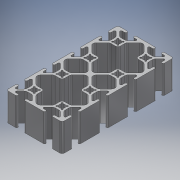
# Autodesk Inventor part: 2040-S
Saved by Autodesk Inventor 2017 SP1 (Build 210196100, 196)
## iProperties
Created: 2016-09-13
Part Number: 2040-S
Material: 6105-T5
Description: 40 S SHORT SINGLE UNIBEARING ASSEMBLY ON 40-4040 X 75mm
Document SubType Name: Modeling
Designer: BRALEF
Density: 1 g/cm^3
Appearance: CLEAR ANODIZED
MATERIAL: 6061-T6
PART PRICE: 44.65
Author: BRALEF
Autodesk Inventor part; units mm, degrees
ref_plane "YZ Plane" through (0, 0, 0) normal (1, 0, 0) x (0, 1, 0)
ref_plane "XZ Plane" through (0, 0, 0) normal (0, 1, 0) x (-1, 0, 0)
ref_plane "XY Plane" through (0, 0, 0) normal (0, 0, 1) x (1, 0, 0)
sketch "Sketch1" plane through (0, 0, 0) normal (0, 1, 0) x (-1, 0, 0)
  arc A0 (-10.6413, -41.7213) -> (-14.7587, -41.7213) centre (-12.7, -43.78) ccw
  line L0 (-19.9529, -46.9156) -> (-14.7587, -41.7213)
  arc A1 (-19.9529, -46.9156) -> (-20.8828, -49.1606) centre (-17.7078, -49.1606) ccw
  line L1 (-20.8828, -53.1074) -> (-20.8828, -49.1606)
  arc A2 (-23.0926, -55.3172) -> (-20.8828, -53.1074) centre (-23.0926, -53.1074) ccw
  line L2 (-27.0394, -55.3172) -> (-23.0926, -55.3172)
  arc A3 (-27.0394, -55.3172) -> (-29.2844, -56.2471) centre (-27.0394, -58.4922) ccw
  line L3 (-34.4787, -61.4413) -> (-29.2844, -56.2471)
  arc A4 (-34.4787, -61.4413) -> (-34.4787, -65.5587) centre (-32.42, -63.5) ccw
  line L4 (-29.2844, -70.7529) -> (-34.4787, -65.5587)
  arc A5 (-29.2844, -70.7529) -> (-27.0394, -71.6828) centre (-27.0394, -68.5078) ccw
  line L5 (-23.0926, -71.6828) -> (-27.0394, -71.6828)
  arc A6 (-20.8828, -73.8926) -> (-23.0926, -71.6828) centre (-23.0926, -73.8926) ccw
  line L6 (-20.8828, -77.8394) -> (-20.8828, -73.8926)
  arc A7 (-20.8828, -77.8394) -> (-19.9529, -80.0844) centre (-17.7078, -77.8394) ccw
  line L7 (-14.7587, -85.2787) -> (-19.9529, -80.0844)
  arc A8 (-14.7587, -85.2787) -> (-10.6413, -85.2787) centre (-12.7, -83.22) ccw
  line L8 (-5.4471, -80.0844) -> (-10.6413, -85.2787)
  arc A9 (-5.4471, -80.0844) -> (-4.5172, -77.8394) centre (-7.6922, -77.8394) ccw
  line L9 (-4.5172, -73.8926) -> (-4.5172, -77.8394)
  arc A10 (-2.3074, -71.6828) -> (-4.5172, -73.8926) centre (-2.3074, -73.8926) ccw
  line L10 (1.6394, -71.6828) -> (-2.3074, -71.6828)
  arc A11 (1.6394, -71.6828) -> (3.8844, -70.7529) centre (1.6394, -68.5078) ccw
  line L11 (9.0787, -65.5587) -> (3.8844, -70.7529)
  arc A12 (9.0787, -65.5587) -> (9.0787, -61.4413) centre (7.02, -63.5) ccw
  line L12 (3.8844, -56.2471) -> (9.0787, -61.4413)
  arc A13 (3.8844, -56.2471) -> (1.6394, -55.3172) centre (1.6394, -58.4922) ccw
  line L13 (-2.3074, -55.3172) -> (1.6394, -55.3172)
  arc A14 (-4.5172, -53.1074) -> (-2.3074, -55.3172) centre (-2.3074, -53.1074) ccw
  line L14 (-4.5172, -49.1606) -> (-4.5172, -53.1074)
  arc A15 (-4.5172, -49.1606) -> (-5.4471, -46.9156) centre (-7.6922, -49.1606) ccw
  line L15 (-10.6413, -41.7213) -> (-5.4471, -46.9156)
  arc A16 (-9.0785, -36.041) -> (-9.0785, -40.159) centre (-7.0195, -38.1) ccw
  line L16 (-3.8846, -45.3529) -> (-9.0785, -40.159)
  arc A17 (-3.8846, -45.3529) -> (-1.6396, -46.2828) centre (-1.6396, -43.1078) ccw
  line L17 (1.6396, -46.2828) -> (-1.6396, -46.2828)
  arc A18 (1.6396, -46.2828) -> (3.8846, -45.3529) centre (1.6396, -43.1078) ccw
  line L18 (9.0785, -40.159) -> (3.8846, -45.3529)
  arc A19 (9.0785, -40.159) -> (9.0785, -36.041) centre (7.0195, -38.1) ccw
  line L19 (3.8846, -30.8471) -> (9.0785, -36.041)
  arc A20 (3.8846, -30.8471) -> (1.6396, -29.9172) centre (1.6396, -33.0922) ccw
  line L20 (-1.6396, -29.9172) -> (1.6396, -29.9172)
  arc A21 (-1.6396, -29.9172) -> (-3.8846, -30.8471) centre (-1.6396, -33.0922) ccw
  line L21 (-9.0785, -36.041) -> (-3.8846, -30.8471)
  arc A22 (-27.3692, -73.3395) -> (-28.2605, -74.2308) centre (-27.8696, -73.7304) ccw
  line L22 (-27.6319, -74.8595) -> (-28.2605, -74.2308)
  arc A23 (-27.6319, -74.8595) -> (-27.6319, -77.5405) centre (-25.4, -76.2) ccw
  line L23 (-28.2605, -78.1692) -> (-27.6319, -77.5405)
  arc A24 (-28.2605, -78.1692) -> (-27.3692, -79.0605) centre (-27.8696, -78.6696) ccw
  line L24 (-26.7405, -78.4319) -> (-27.3692, -79.0605)
  arc A25 (-26.7405, -78.4319) -> (-24.0595, -78.4319) centre (-25.4, -76.2) ccw
  line L25 (-23.4308, -79.0605) -> (-24.0595, -78.4319)
  arc A26 (-23.4308, -79.0605) -> (-22.5395, -78.1692) centre (-22.9304, -78.6696) ccw
  line L26 (-23.1681, -77.5405) -> (-22.5395, -78.1692)
  arc A27 (-23.1681, -77.5405) -> (-23.1681, -74.8595) centre (-25.4, -76.2) ccw
  line L27 (-22.5395, -74.2308) -> (-23.1681, -74.8595)
  arc A28 (-22.5395, -74.2308) -> (-23.4308, -73.3395) centre (-22.9304, -73.7304) ccw
  line L28 (-24.0595, -73.9681) -> (-23.4308, -73.3395)
  arc A29 (-24.0595, -73.9681) -> (-26.7405, -73.9681) centre (-25.4, -76.2) ccw
  line L29 (-27.3692, -73.3395) -> (-26.7405, -73.9681)
  arc A30 (-27.3692, -47.9395) -> (-28.2605, -48.8308) centre (-27.8696, -48.3304) ccw
  line L30 (-27.6319, -49.4595) -> (-28.2605, -48.8308)
  arc A31 (-27.6319, -49.4595) -> (-27.6319, -52.1405) centre (-25.4, -50.8) ccw
  line L31 (-28.2605, -52.7692) -> (-27.6319, -52.1405)
  arc A32 (-28.2605, -52.7692) -> (-27.3692, -53.6605) centre (-27.8696, -53.2696) ccw
  line L32 (-26.7405, -53.0319) -> (-27.3692, -53.6605)
  arc A33 (-26.7405, -53.0319) -> (-24.0595, -53.0319) centre (-25.4, -50.8) ccw
  line L33 (-23.4308, -53.6605) -> (-24.0595, -53.0319)
  arc A34 (-23.4308, -53.6605) -> (-22.5395, -52.7692) centre (-22.9304, -53.2696) ccw
  line L34 (-23.1681, -52.1405) -> (-22.5395, -52.7692)
  arc A35 (-23.1681, -52.1405) -> (-23.1681, -49.4595) centre (-25.4, -50.8) ccw
  line L35 (-22.5395, -48.8308) -> (-23.1681, -49.4595)
  arc A36 (-22.5395, -48.8308) -> (-23.4308, -47.9395) centre (-22.9304, -48.3304) ccw
  line L36 (-24.0595, -48.5681) -> (-23.4308, -47.9395)
  arc A37 (-24.0595, -48.5681) -> (-26.7405, -48.5681) centre (-25.4, -50.8) ccw
  line L37 (-27.3692, -47.9395) -> (-26.7405, -48.5681)
  arc A38 (-1.9692, -22.5395) -> (-2.8605, -23.4308) centre (-2.4696, -22.9304) ccw
  line L38 (-2.2319, -24.0595) -> (-2.8605, -23.4308)
  arc A39 (-2.2319, -24.0595) -> (-2.2319, -26.7405) centre (0, -25.4) ccw
  line L39 (-2.8605, -27.3692) -> (-2.2319, -26.7405)
  arc A40 (-2.8605, -27.3692) -> (-1.9692, -28.2605) centre (-2.4696, -27.8696) ccw
  line L40 (-1.3405, -27.6319) -> (-1.9692, -28.2605)
  arc A41 (-1.3405, -27.6319) -> (1.3405, -27.6319) centre (0, -25.4) ccw
  line L41 (1.9692, -28.2605) -> (1.3405, -27.6319)
  arc A42 (1.9692, -28.2605) -> (2.8605, -27.3692) centre (2.4696, -27.8696) ccw
  line L42 (2.2319, -26.7405) -> (2.8605, -27.3692)
  arc A43 (2.2319, -26.7405) -> (2.2319, -24.0595) centre (0, -25.4) ccw
  line L43 (2.8605, -23.4308) -> (2.2319, -24.0595)
  arc A44 (2.8605, -23.4308) -> (1.9692, -22.5395) centre (2.4696, -22.9304) ccw
  line L44 (1.3405, -23.1681) -> (1.9692, -22.5395)
  arc A45 (1.3405, -23.1681) -> (-1.3405, -23.1681) centre (0, -25.4) ccw
  line L45 (-1.9692, -22.5395) -> (-1.3405, -23.1681)
  arc A46 (-1.9692, 2.8605) -> (-2.8605, 1.9692) centre (-2.4696, 2.4696) ccw
  line L46 (-2.2319, 1.3405) -> (-2.8605, 1.9692)
  arc A47 (-2.2319, 1.3405) -> (-2.2319, -1.3405) centre (0, 0) ccw
  line L47 (-2.8605, -1.9692) -> (-2.2319, -1.3405)
  arc A48 (-2.8605, -1.9692) -> (-1.9692, -2.8605) centre (-2.4696, -2.4696) ccw
  line L48 (-1.3405, -2.2319) -> (-1.9692, -2.8605)
  arc A49 (-1.3405, -2.2319) -> (1.3405, -2.2319) centre (0, 0) ccw
  line L49 (1.9692, -2.8605) -> (1.3405, -2.2319)
  arc A50 (1.9692, -2.8605) -> (2.8605, -1.9692) centre (2.4696, -2.4696) ccw
  line L50 (2.2319, -1.3405) -> (2.8605, -1.9692)
  arc A51 (2.2319, -1.3405) -> (2.2319, 1.3405) centre (0, 0) ccw
  line L51 (2.8605, 1.9692) -> (2.2319, 1.3405)
  arc A52 (2.8605, 1.9692) -> (1.9692, 2.8605) centre (2.4696, 2.4696) ccw
  line L52 (1.3405, 2.2319) -> (1.9692, 2.8605)
  arc A53 (1.3405, 2.2319) -> (-1.3405, 2.2319) centre (0, 0) ccw
  line L53 (-1.9692, 2.8605) -> (-1.3405, 2.2319)
  arc A54 (-1.3405, -53.0319) -> (1.3405, -53.0319) centre (0, -50.8) ccw
  line L54 (1.9692, -53.6605) -> (1.3405, -53.0319)
  arc A55 (1.9692, -53.6605) -> (2.8605, -52.7692) centre (2.4696, -53.2696) ccw
  line L55 (2.2319, -52.1405) -> (2.8605, -52.7692)
  arc A56 (2.2319, -52.1405) -> (2.2319, -49.4595) centre (0, -50.8) ccw
  line L56 (2.8605, -48.8308) -> (2.2319, -49.4595)
  arc A57 (2.8605, -48.8308) -> (1.9692, -47.9395) centre (2.4696, -48.3304) ccw
  line L57 (1.3405, -48.5681) -> (1.9692, -47.9395)
  arc A58 (1.3405, -48.5681) -> (-1.3405, -48.5681) centre (0, -50.8) ccw
  line L58 (-1.9692, -47.9395) -> (-1.3405, -48.5681)
  arc A59 (-1.9692, -47.9395) -> (-2.8605, -48.8308) centre (-2.4696, -48.3304) ccw
  line L59 (-2.2319, -49.4595) -> (-2.8605, -48.8308)
  arc A60 (-2.2319, -49.4595) -> (-2.2319, -52.1405) centre (0, -50.8) ccw
  line L60 (-2.8605, -52.7692) -> (-2.2319, -52.1405)
  arc A61 (-2.8605, -52.7692) -> (-1.9692, -53.6605) centre (-2.4696, -53.2696) ccw
  line L61 (-1.3405, -53.0319) -> (-1.9692, -53.6605)
  arc A62 (-27.3692, 2.8605) -> (-28.2605, 1.9692) centre (-27.8696, 2.4696) ccw
  line L62 (-27.6319, 1.3405) -> (-28.2605, 1.9692)
  arc A63 (-27.6319, 1.3405) -> (-27.6319, -1.3405) centre (-25.4, 0) ccw
  line L63 (-28.2605, -1.9692) -> (-27.6319, -1.3405)
  arc A64 (-28.2605, -1.9692) -> (-27.3692, -2.8605) centre (-27.8696, -2.4696) ccw
  line L64 (-26.7405, -2.2319) -> (-27.3692, -2.8605)
  arc A65 (-26.7405, -2.2319) -> (-24.0595, -2.2319) centre (-25.4, 0) ccw
  line L65 (-23.4308, -2.8605) -> (-24.0595, -2.2319)
  arc A66 (-23.4308, -2.8605) -> (-22.5395, -1.9692) centre (-22.9304, -2.4696) ccw
  line L66 (-23.1681, -1.3405) -> (-22.5395, -1.9692)
  arc A67 (-23.1681, -1.3405) -> (-23.1681, 1.3405) centre (-25.4, 0) ccw
  line L67 (-22.5395, 1.9692) -> (-23.1681, 1.3405)
  arc A68 (-22.5395, 1.9692) -> (-23.4308, 2.8605) centre (-22.9304, 2.4696) ccw
  line L68 (-24.0595, 2.2319) -> (-23.4308, 2.8605)
  arc A69 (-24.0595, 2.2319) -> (-26.7405, 2.2319) centre (-25.4, 0) ccw
  line L69 (-27.3692, 2.8605) -> (-26.7405, 2.2319)
  arc A70 (-27.3692, -22.5395) -> (-28.2605, -23.4308) centre (-27.8696, -22.9304) ccw
  line L70 (-27.6319, -24.0595) -> (-28.2605, -23.4308)
  arc A71 (-27.6319, -24.0595) -> (-27.6319, -26.7405) centre (-25.4, -25.4) ccw
  line L71 (-28.2605, -27.3692) -> (-27.6319, -26.7405)
  arc A72 (-28.2605, -27.3692) -> (-27.3692, -28.2605) centre (-27.8696, -27.8696) ccw
  line L72 (-26.7405, -27.6319) -> (-27.3692, -28.2605)
  arc A73 (-26.7405, -27.6319) -> (-24.0595, -27.6319) centre (-25.4, -25.4) ccw
  line L73 (-23.4308, -28.2605) -> (-24.0595, -27.6319)
  arc A74 (-23.4308, -28.2605) -> (-22.5395, -27.3692) centre (-22.9304, -27.8696) ccw
  line L74 (-23.1681, -26.7405) -> (-22.5395, -27.3692)
  arc A75 (-23.1681, -26.7405) -> (-23.1681, -24.0595) centre (-25.4, -25.4) ccw
  line L75 (-22.5395, -23.4308) -> (-23.1681, -24.0595)
  arc A76 (-22.5395, -23.4308) -> (-23.4308, -22.5395) centre (-22.9304, -22.9304) ccw
  line L76 (-24.0595, -23.1681) -> (-23.4308, -22.5395)
  arc A77 (-24.0595, -23.1681) -> (-26.7405, -23.1681) centre (-25.4, -25.4) ccw
  line L77 (-27.3692, -22.5395) -> (-26.7405, -23.1681)
  arc A78 (-1.9692, -73.3395) -> (-2.8605, -74.2308) centre (-2.4696, -73.7304) ccw
  line L78 (-2.2319, -74.8595) -> (-2.8605, -74.2308)
  arc A79 (-2.2319, -74.8595) -> (-2.2319, -77.5405) centre (0, -76.2) ccw
  line L79 (-2.8605, -78.1692) -> (-2.2319, -77.5405)
  arc A80 (-2.8605, -78.1692) -> (-1.9692, -79.0605) centre (-2.4696, -78.6696) ccw
  line L80 (-1.3405, -78.4319) -> (-1.9692, -79.0605)
  arc A81 (-1.3405, -78.4319) -> (1.3405, -78.4319) centre (0, -76.2) ccw
  line L81 (1.9692, -79.0605) -> (1.3405, -78.4319)
  arc A82 (1.9692, -79.0605) -> (2.8605, -78.1692) centre (2.4696, -78.6696) ccw
  line L82 (2.2319, -77.5405) -> (2.8605, -78.1692)
  arc A83 (2.2319, -77.5405) -> (2.2319, -74.8595) centre (0, -76.2) ccw
  line L83 (2.8605, -74.2308) -> (2.2319, -74.8595)
  arc A84 (2.8605, -74.2308) -> (1.9692, -73.3395) centre (2.4696, -73.7304) ccw
  line L84 (1.3405, -73.9681) -> (1.9692, -73.3395)
  arc A85 (1.3405, -73.9681) -> (-1.3405, -73.9681) centre (0, -76.2) ccw
  line L85 (-1.9692, -73.3395) -> (-1.3405, -73.9681)
  arc A86 (-34.4785, -36.041) -> (-34.4785, -40.159) centre (-32.4195, -38.1) ccw
  line L86 (-29.2846, -45.3529) -> (-34.4785, -40.159)
  arc A87 (-29.2846, -45.3529) -> (-27.0396, -46.2828) centre (-27.0396, -43.1078) ccw
  line L87 (-23.7604, -46.2828) -> (-27.0396, -46.2828)
  arc A88 (-23.7604, -46.2828) -> (-21.5154, -45.3529) centre (-23.7604, -43.1078) ccw
  line L88 (-16.3215, -40.159) -> (-21.5154, -45.3529)
  arc A89 (-16.3215, -40.159) -> (-16.3215, -36.041) centre (-18.3805, -38.1) ccw
  line L89 (-21.5154, -30.8471) -> (-16.3215, -36.041)
  arc A90 (-21.5154, -30.8471) -> (-23.7604, -29.9172) centre (-23.7604, -33.0922) ccw
  line L90 (-27.0396, -29.9172) -> (-23.7604, -29.9172)
  arc A91 (-27.0396, -29.9172) -> (-29.2846, -30.8471) centre (-27.0396, -33.0922) ccw
  line L91 (-34.4785, -36.041) -> (-29.2846, -30.8471)
  arc A92 (-10.6413, 9.0787) -> (-14.7587, 9.0787) centre (-12.7, 7.02) ccw
  line L92 (-19.9529, 3.8844) -> (-14.7587, 9.0787)
  arc A93 (-19.9529, 3.8844) -> (-20.8828, 1.6394) centre (-17.7078, 1.6394) ccw
  line L93 (-20.8828, -2.3074) -> (-20.8828, 1.6394)
  arc A94 (-23.0926, -4.5172) -> (-20.8828, -2.3074) centre (-23.0926, -2.3074) ccw
  line L94 (-27.0394, -4.5172) -> (-23.0926, -4.5172)
  arc A95 (-27.0394, -4.5172) -> (-29.2844, -5.4471) centre (-27.0394, -7.6922) ccw
  line L95 (-34.4787, -10.6413) -> (-29.2844, -5.4471)
  arc A96 (-34.4787, -10.6413) -> (-34.4787, -14.7587) centre (-32.42, -12.7) ccw
  line L96 (-29.2844, -19.9529) -> (-34.4787, -14.7587)
  arc A97 (-29.2844, -19.9529) -> (-27.0394, -20.8828) centre (-27.0394, -17.7078) ccw
  line L97 (-23.0926, -20.8828) -> (-27.0394, -20.8828)
  arc A98 (-20.8828, -23.0926) -> (-23.0926, -20.8828) centre (-23.0926, -23.0926) ccw
  line L98 (-20.8828, -27.0394) -> (-20.8828, -23.0926)
  arc A99 (-20.8828, -27.0394) -> (-19.9529, -29.2844) centre (-17.7078, -27.0394) ccw
  line L99 (-14.7587, -34.4787) -> (-19.9529, -29.2844)
  arc A100 (-14.7587, -34.4787) -> (-10.6413, -34.4787) centre (-12.7, -32.42) ccw
  line L100 (-5.4471, -29.2844) -> (-10.6413, -34.4787)
  arc A101 (-5.4471, -29.2844) -> (-4.5172, -27.0394) centre (-7.6922, -27.0394) ccw
  line L101 (-4.5172, -23.0926) -> (-4.5172, -27.0394)
  arc A102 (-2.3074, -20.8828) -> (-4.5172, -23.0926) centre (-2.3074, -23.0926) ccw
  line L102 (1.6394, -20.8828) -> (-2.3074, -20.8828)
  arc A103 (1.6394, -20.8828) -> (3.8844, -19.9529) centre (1.6394, -17.7078) ccw
  line L103 (9.0787, -14.7587) -> (3.8844, -19.9529)
  arc A104 (9.0787, -14.7587) -> (9.0787, -10.6413) centre (7.02, -12.7) ccw
  line L104 (3.8844, -5.4471) -> (9.0787, -10.6413)
  arc A105 (3.8844, -5.4471) -> (1.6394, -4.5172) centre (1.6394, -7.6922) ccw
  line L105 (-2.3074, -4.5172) -> (1.6394, -4.5172)
  arc A106 (-4.5172, -2.3074) -> (-2.3074, -4.5172) centre (-2.3074, -2.3074) ccw
  line L106 (-4.5172, 1.6394) -> (-4.5172, -2.3074)
  arc A107 (-4.5172, 1.6394) -> (-5.4471, 3.8844) centre (-7.6922, 1.6394) ccw
  line L107 (-10.6413, 9.0787) -> (-5.4471, 3.8844)
  arc A108 (12.7, -29.7561) -> (10.4902, -29.7561) centre (11.5951, -29.7561) ccw
  line L108 (12.7, -29.7561) -> (12.7, -46.4439)
  arc A109 (10.4902, -46.4439) -> (12.7, -46.4439) centre (11.5951, -46.4439) ccw
  line L109 (10.4902, -46.4439) -> (10.4902, -44.3251)
  arc A110 (10.4902, -44.3251) -> (8.7558, -43.6067) centre (9.4742, -44.3251) ccw
  line L110 (8.7558, -43.6067) -> (5.4471, -46.9154)
  arc A111 (5.4471, -46.9154) -> (4.5172, -49.1604) centre (7.6922, -49.1604) ccw
  line L111 (4.5172, -49.1604) -> (4.5172, -52.4396)
  arc A112 (4.5172, -52.4396) -> (5.4471, -54.6846) centre (7.6922, -52.4396) ccw
  line L112 (5.4471, -54.6846) -> (8.7558, -57.9933)
  arc A113 (8.7558, -57.9933) -> (10.4902, -57.2749) centre (9.4742, -57.2749) ccw
  line L113 (10.4902, -57.2749) -> (10.4902, -55.1561)
  arc A114 (12.7, -55.1561) -> (10.4902, -55.1561) centre (11.5951, -55.1561) ccw
  line L114 (12.7, -55.1561) -> (12.7, -71.8439)
  arc A115 (10.4902, -71.8439) -> (12.7, -71.8439) centre (11.5951, -71.8439) ccw
  line L115 (10.4902, -71.8439) -> (10.4902, -69.7251)
  arc A116 (10.4902, -69.7251) -> (8.7558, -69.0067) centre (9.4742, -69.7251) ccw
  line L116 (8.7558, -69.0067) -> (5.4471, -72.3154)
  arc A117 (5.4471, -72.3154) -> (4.5172, -74.5604) centre (7.6922, -74.5604) ccw
  line L117 (4.5172, -74.5604) -> (4.5172, -77.8396)
  arc A118 (4.5172, -77.8396) -> (5.4471, -80.0846) centre (7.6922, -77.8396) ccw
  line L118 (5.4471, -80.0846) -> (8.7558, -83.3933)
  arc A119 (8.7558, -83.3933) -> (10.4902, -82.6749) centre (9.4742, -82.6749) ccw
  line L119 (10.4902, -82.6749) -> (10.4902, -80.5561)
  arc A120 (12.7, -80.5561) -> (10.4902, -80.5561) centre (11.5951, -80.5561) ccw
  line L120 (12.7, -80.5561) -> (12.7, -86.7918)
  arc A121 (10.5918, -88.9) -> (12.7, -86.7918) centre (10.5918, -86.7918) ccw
  line L121 (10.5918, -88.9) -> (4.3561, -88.9)
  arc A122 (4.3561, -86.6902) -> (4.3561, -88.9) centre (4.3561, -87.7951) ccw
  line L122 (4.3561, -86.6902) -> (6.4749, -86.6902)
  arc A123 (6.4749, -86.6902) -> (7.1933, -84.9558) centre (6.4749, -85.6742) ccw
  line L123 (7.1933, -84.9558) -> (3.8846, -81.6471)
  arc A124 (3.8846, -81.6471) -> (1.6396, -80.7172) centre (1.6396, -83.8922) ccw
  line L124 (1.6396, -80.7172) -> (-1.6396, -80.7172)
  arc A125 (-1.6396, -80.7172) -> (-3.8846, -81.6471) centre (-1.6396, -83.8922) ccw
  line L125 (-3.8846, -81.6471) -> (-7.1933, -84.9558)
  arc A126 (-7.1933, -84.9558) -> (-6.4749, -86.6902) centre (-6.4749, -85.6742) ccw
  line L126 (-6.4749, -86.6902) -> (-4.3561, -86.6902)
  arc A127 (-4.3561, -88.9) -> (-4.3561, -86.6902) centre (-4.3561, -87.7951) ccw
  line L127 (-4.3561, -88.9) -> (-21.0439, -88.9)
  arc A128 (-21.0439, -86.6902) -> (-21.0439, -88.9) centre (-21.0439, -87.7951) ccw
  line L128 (-21.0439, -86.6902) -> (-18.9251, -86.6902)
  arc A129 (-18.9251, -86.6902) -> (-18.2067, -84.9558) centre (-18.9251, -85.6742) ccw
  line L129 (-18.2067, -84.9558) -> (-21.5154, -81.6471)
  arc A130 (-21.5154, -81.6471) -> (-23.7604, -80.7172) centre (-23.7604, -83.8922) ccw
  line L130 (-23.7604, -80.7172) -> (-27.0396, -80.7172)
  arc A131 (-27.0396, -80.7172) -> (-29.2846, -81.6471) centre (-27.0396, -83.8922) ccw
  line L131 (-29.2846, -81.6471) -> (-32.5933, -84.9558)
  arc A132 (-32.5933, -84.9558) -> (-31.8749, -86.6902) centre (-31.8749, -85.6742) ccw
  line L132 (-31.8749, -86.6902) -> (-29.7561, -86.6902)
  arc A133 (-29.7561, -88.9) -> (-29.7561, -86.6902) centre (-29.7561, -87.7951) ccw
  line L133 (-29.7561, -88.9) -> (-35.9918, -88.9)
  arc A134 (-38.1, -86.7918) -> (-35.9918, -88.9) centre (-35.9918, -86.7918) ccw
  line L134 (-38.1, -86.7918) -> (-38.1, -80.5561)
  arc A135 (-35.8902, -80.5561) -> (-38.1, -80.5561) centre (-36.9951, -80.5561) ccw
  line L135 (-35.8902, -80.5561) -> (-35.8902, -82.6749)
  arc A136 (-35.8902, -82.6749) -> (-34.1558, -83.3933) centre (-34.8742, -82.6749) ccw
  line L136 (-34.1558, -83.3933) -> (-30.8471, -80.0846)
  arc A137 (-30.8471, -80.0846) -> (-29.9172, -77.8396) centre (-33.0922, -77.8396) ccw
  line L137 (-29.9172, -77.8396) -> (-29.9172, -74.5604)
  arc A138 (-29.9172, -74.5604) -> (-30.8471, -72.3154) centre (-33.0922, -74.5604) ccw
  line L138 (-30.8471, -72.3154) -> (-34.1558, -69.0067)
  arc A139 (-34.1558, -69.0067) -> (-35.8902, -69.7251) centre (-34.8742, -69.7251) ccw
  line L139 (-35.8902, -69.7251) -> (-35.8902, -71.8439)
  arc A140 (-38.1, -71.8439) -> (-35.8902, -71.8439) centre (-36.9951, -71.8439) ccw
  line L140 (-38.1, -71.8439) -> (-38.1, -55.1561)
  arc A141 (-35.8902, -55.1561) -> (-38.1, -55.1561) centre (-36.9951, -55.1561) ccw
  line L141 (-35.8902, -55.1561) -> (-35.8902, -57.2749)
  arc A142 (-35.8902, -57.2749) -> (-34.1558, -57.9933) centre (-34.8742, -57.2749) ccw
  line L142 (-34.1558, -57.9933) -> (-30.8471, -54.6846)
  arc A143 (-30.8471, -54.6846) -> (-29.9172, -52.4396) centre (-33.0922, -52.4396) ccw
  line L143 (-29.9172, -52.4396) -> (-29.9172, -49.1604)
  arc A144 (-29.9172, -49.1604) -> (-30.8471, -46.9154) centre (-33.0922, -49.1604) ccw
  line L144 (-30.8471, -46.9154) -> (-34.1558, -43.6067)
  arc A145 (-34.1558, -43.6067) -> (-35.8902, -44.3251) centre (-34.8742, -44.3251) ccw
  line L145 (-35.8902, -44.3251) -> (-35.8902, -46.4439)
  arc A146 (-38.1, -46.4439) -> (-35.8902, -46.4439) centre (-36.9951, -46.4439) ccw
  line L146 (-38.1, -46.4439) -> (-38.1, -29.7561)
  arc A147 (-35.8902, -29.7561) -> (-38.1, -29.7561) centre (-36.9951, -29.7561) ccw
  line L147 (-35.8902, -29.7561) -> (-35.8902, -31.8749)
  arc A148 (-35.8902, -31.8749) -> (-34.1558, -32.5933) centre (-34.8742, -31.8749) ccw
  line L148 (-34.1558, -32.5933) -> (-30.8471, -29.2846)
  arc A149 (-30.8471, -29.2846) -> (-29.9172, -27.0396) centre (-33.0922, -27.0396) ccw
  line L149 (-29.9172, -27.0396) -> (-29.9172, -23.7604)
  arc A150 (-29.9172, -23.7604) -> (-30.8471, -21.5154) centre (-33.0922, -23.7604) ccw
  line L150 (-30.8471, -21.5154) -> (-34.1558, -18.2067)
  arc A151 (-34.1558, -18.2067) -> (-35.8902, -18.9251) centre (-34.8742, -18.9251) ccw
  line L151 (-35.8902, -18.9251) -> (-35.8902, -21.0439)
  arc A152 (-38.1, -21.0439) -> (-35.8902, -21.0439) centre (-36.9951, -21.0439) ccw
  line L152 (-38.1, -21.0439) -> (-38.1, -4.3561)
  arc A153 (-35.8902, -4.3561) -> (-38.1, -4.3561) centre (-36.9951, -4.3561) ccw
  line L153 (-35.8902, -4.3561) -> (-35.8902, -6.4749)
  arc A154 (-35.8902, -6.4749) -> (-34.1558, -7.1933) centre (-34.8742, -6.4749) ccw
  line L154 (-34.1558, -7.1933) -> (-30.8471, -3.8846)
  arc A155 (-30.8471, -3.8846) -> (-29.9172, -1.6396) centre (-33.0922, -1.6396) ccw
  line L155 (-29.9172, -1.6396) -> (-29.9172, 1.6396)
  arc A156 (-29.9172, 1.6396) -> (-30.8471, 3.8846) centre (-33.0922, 1.6396) ccw
  line L156 (-30.8471, 3.8846) -> (-34.1558, 7.1933)
  arc A157 (-34.1558, 7.1933) -> (-35.8902, 6.4749) centre (-34.8742, 6.4749) ccw
  line L157 (-35.8902, 6.4749) -> (-35.8902, 4.3561)
  arc A158 (-38.1, 4.3561) -> (-35.8902, 4.3561) centre (-36.9951, 4.3561) ccw
  line L158 (-38.1, 4.3561) -> (-38.1, 10.5918)
  arc A159 (-35.9918, 12.7) -> (-38.1, 10.5918) centre (-35.9918, 10.5918) ccw
  line L159 (-35.9918, 12.7) -> (-29.7561, 12.7)
  arc A160 (-29.7561, 10.4902) -> (-29.7561, 12.7) centre (-29.7561, 11.5951) ccw
  line L160 (-29.7561, 10.4902) -> (-31.8749, 10.4902)
  arc A161 (-31.8749, 10.4902) -> (-32.5933, 8.7558) centre (-31.8749, 9.4742) ccw
  line L161 (-32.5933, 8.7558) -> (-29.2846, 5.4471)
  arc A162 (-29.2846, 5.4471) -> (-27.0396, 4.5172) centre (-27.0396, 7.6922) ccw
  line L162 (-27.0396, 4.5172) -> (-23.7604, 4.5172)
  arc A163 (-23.7604, 4.5172) -> (-21.5154, 5.4471) centre (-23.7604, 7.6922) ccw
  line L163 (-21.5154, 5.4471) -> (-18.2067, 8.7558)
  arc A164 (-18.2067, 8.7558) -> (-18.9251, 10.4902) centre (-18.9251, 9.4742) ccw
  line L164 (-18.9251, 10.4902) -> (-21.0439, 10.4902)
  arc A165 (-21.0439, 12.7) -> (-21.0439, 10.4902) centre (-21.0439, 11.5951) ccw
  line L165 (-21.0439, 12.7) -> (-4.3561, 12.7)
  arc A166 (-4.3561, 10.4902) -> (-4.3561, 12.7) centre (-4.3561, 11.5951) ccw
  line L166 (-4.3561, 10.4902) -> (-6.4749, 10.4902)
  arc A167 (-6.4749, 10.4902) -> (-7.1933, 8.7558) centre (-6.4749, 9.4742) ccw
  line L167 (-7.1933, 8.7558) -> (-3.8846, 5.4471)
  arc A168 (-3.8846, 5.4471) -> (-1.6396, 4.5172) centre (-1.6396, 7.6922) ccw
  line L168 (-1.6396, 4.5172) -> (1.6396, 4.5172)
  arc A169 (1.6396, 4.5172) -> (3.8846, 5.4471) centre (1.6396, 7.6922) ccw
  line L169 (3.8846, 5.4471) -> (7.1933, 8.7558)
  arc A170 (7.1933, 8.7558) -> (6.4749, 10.4902) centre (6.4749, 9.4742) ccw
  line L170 (6.4749, 10.4902) -> (4.3561, 10.4902)
  arc A171 (4.3561, 12.7) -> (4.3561, 10.4902) centre (4.3561, 11.5951) ccw
  line L171 (4.3561, 12.7) -> (10.5918, 12.7)
  arc A172 (12.7, 10.5918) -> (10.5918, 12.7) centre (10.5918, 10.5918) ccw
  line L172 (12.7, 10.5918) -> (12.7, 4.3561)
  arc A173 (10.4902, 4.3561) -> (12.7, 4.3561) centre (11.5951, 4.3561) ccw
  line L173 (10.4902, 4.3561) -> (10.4902, 6.4749)
  arc A174 (10.4902, 6.4749) -> (8.7558, 7.1933) centre (9.4742, 6.4749) ccw
  line L174 (8.7558, 7.1933) -> (5.4471, 3.8846)
  arc A175 (5.4471, 3.8846) -> (4.5172, 1.6396) centre (7.6922, 1.6396) ccw
  line L175 (4.5172, 1.6396) -> (4.5172, -1.6396)
  arc A176 (4.5172, -1.6396) -> (5.4471, -3.8846) centre (7.6922, -1.6396) ccw
  line L176 (5.4471, -3.8846) -> (8.7558, -7.1933)
  arc A177 (8.7558, -7.1933) -> (10.4902, -6.4749) centre (9.4742, -6.4749) ccw
  line L177 (10.4902, -6.4749) -> (10.4902, -4.3561)
  arc A178 (12.7, -4.3561) -> (10.4902, -4.3561) centre (11.5951, -4.3561) ccw
  line L178 (12.7, -4.3561) -> (12.7, -21.0439)
  arc A179 (10.4902, -21.0439) -> (12.7, -21.0439) centre (11.5951, -21.0439) ccw
  line L179 (10.4902, -21.0439) -> (10.4902, -18.9251)
  arc A180 (10.4902, -18.9251) -> (8.7558, -18.2067) centre (9.4742, -18.9251) ccw
  line L180 (8.7558, -18.2067) -> (5.4471, -21.5154)
  arc A181 (5.4471, -21.5154) -> (4.5172, -23.7604) centre (7.6922, -23.7604) ccw
  line L181 (4.5172, -23.7604) -> (4.5172, -27.0396)
  arc A182 (4.5172, -27.0396) -> (5.4471, -29.2846) centre (7.6922, -27.0396) ccw
  line L182 (5.4471, -29.2846) -> (8.7558, -32.5933)
  arc A183 (8.7558, -32.5933) -> (10.4902, -31.8749) centre (9.4742, -31.8749) ccw
  line L183 (10.4902, -31.8749) -> (10.4902, -29.7561)
  point P0 (0, 0)
  constraints: 368 end point, 368 point on circle, 184 centre point
extrude "Extrusion1" add sketch "Sketch1" along normal mid plane 25.4
body "Solid1"
